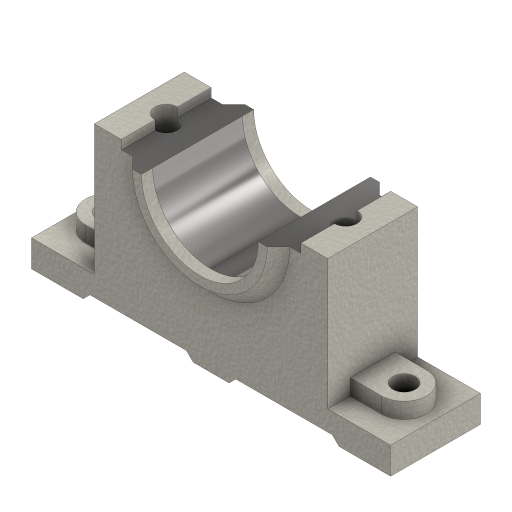
# Autodesk Inventor part: Part039. Lower halg bearing
Saved by Autodesk Inventor 2023.2 (Build 272271030, 271C)
## iProperties
Created: 2023-11-29
Part Number: Part039. Lower halg bearing
Material: Steel, Carbon
Document SubType Name: Modeling
Designer: User
Mass: 237.054 g
Surface Area: 100.472 cm^2
Volume: 30.198 cm^3
Density: 7.85 g/cm^3
Appearance: Steel - Cast
Author: User
Autodesk Inventor part; units mm, degrees
ref_plane "YZ Plane" through (0, 0, 0) normal (1, 0, 0) x (0, 1, 0)
ref_plane "XZ Plane" through (0, 0, 0) normal (0, 1, 0) x (-1, 0, 0)
ref_plane "XY Plane" through (0, 0, 0) normal (0, 0, 1) x (1, 0, 0)
sketch "Sketch1" plane through (0, 0, 0) normal (0, 0, 1) x (1, 0, 0)
  line L0 (0, 0) -> (0, 35) construction
  line L1 (0, 0) -> (-4, 0)
  line L2 (-4, 0) -> (-5.5, 1.5)
  line L3 (-5.5, 1.5) -> (-27, 1.5)
  line L4 (-27, 1.5) -> (-28.5, 0)
  line L5 (-28.5, 0) -> (-40, 0)
  line L6 (-40, 0) -> (-40, 6)
  line L7 (-40, 6) -> (-26, 6)
  line L8 (-26, 6) -> (-26, 35)
  line L9 (-26, 35) -> (-20, 35)
  line L10 (-20, 35) -> (-20, 33)
  line L11 (-20, 33) -> (-13.0111, 33)
  arc A0 (-13.0111, 33) -> (0, 20) centre (-0.0111, 33) ccw
  line L12 (0, 0) -> (4, 0)
  line L13 (4, 0) -> (5.5, 1.5)
  line L14 (5.5, 1.5) -> (27, 1.5)
  line L15 (27, 1.5) -> (28.5, 0)
  line L16 (28.5, 0) -> (40, 0)
  line L17 (40, 0) -> (40, 6)
  line L18 (40, 6) -> (26, 6)
  line L19 (26, 6) -> (26, 35)
  line L20 (26, 35) -> (20, 35)
  line L21 (20, 35) -> (20, 33)
  line L22 (20, 33) -> (13.0111, 33)
  arc A1 (0, 20) -> (13.0111, 33) centre (0.0111, 33) ccw
  dimension "d0" = 35
  dimension "d1" = 45
  dimension "d2" = 45
  dimension "d3" = 24.5
  dimension "d4" = 1.5
  dimension "d5" = 8
  dimension "d6" = 6
  dimension "d7" = 13
  dimension "d8" = 40
  dimension "d9" = 52
  dimension "d10" = 2
  dimension "d11" = 80
  dimension "d12" = 26.9889
  constraints: 46 end point, 12 symmetric about line, 8 point on line, 6 perpendicular, 4 point on circle, 2 centre point, 1 horizontal, 1 parallel, 1 vertical, 1 other
  measures "d0" distance of L0.start L0.end
  measures "d1" angle of L5 L4
  measures "d2" angle of L3 L2
  measures "d3" distance of L1.end L4.end
  measures "d4" distance between parallel lines of L1 L3
  measures "d5" distance of L12.end L1.end
  measures "d6" distance between parallel lines of L16 L18
  measures "d7" radius of A1
  measures "d8" distance between parallel lines of L21 L10
  measures "d9" distance between parallel lines of L19 L8
  measures "d10" distance between parallel lines of L11 L9
  measures "d11" distance between parallel lines of L17 L6
  measures "d12" distance from line of L22.end L17
extrude "Extrusion1" add sketch "Sketch1" along normal mid plane 20
sketch "Sketch2" plane through (26, 6, 10) normal (0, 1, 0) x (1, 0, 0)
  line L0 (0, 20) -> (0, 0) projected
  line L1 (0, 20) -> (0, 0) projected
  line L2 (0, 15) -> (7, 15)
  arc A0 (7, 5) -> (7, 15) centre (7, 10) ccw
  line L3 (7, 5) -> (0, 5)
  line L4 (-26, 20) -> (-26, 0) projected
  point P0 (-26, 10)
  point P1 (-26, 10)
  point P2 (-26, 10)
  dimension "d15" = 5
  dimension "d16" = 33
  constraints: 4 end point, 2 midpoint, 2 point on circle, 2 point on line, 2 tangent, 1 centre point, 1 horizontal, 1 horizontal alignment, 1 parallel
  measures "d15" radius of A0
  measures "d16" distance of point (-26, 10) A0.centre
extrude "Extrusion2" add sketch "Sketch2" along normal blind 3.5
sketch "Sketch3" plane through (26, 9.5, 10) normal (0, 1, 0) x (1, 0, 0)
  arc A0 (7, 5) -> (7, 15) centre (7, 10) ccw projected
  point P0 (-26, 10)
  constraints: 1 coincident
hole "Hole1" at (33, 9.5, 0) direction (0, -1, 0) diameter 5 end through all
mirror "Mirror1" about plane through (0, 0, 0) normal (1, 0, 0) of "Extrusion2", "Hole1"
sketch "Sketch4" plane through (-20, 33, 10) normal (0, 1, 0) x (1, 0, 0)
  line L0 (6.9889, 0) -> (0, 0) projected
  line L1 (6.9889, 0) -> (6.9889, -2.5)
  line L2 (6.9889, -2.5) -> (5, -2.5)
  line L3 (5, -2.5) -> (2.5, 0)
  line L4 (20, 24.7399) -> (20, -8.4394) projected
  point P0 (20, 10)
  dimension "d26" = 30
  dimension "d27" = 45
  dimension "d28" = 12.5
  constraints: 6 end point, 1 perpendicular, 1 point on line, 1 vertical
  measures "d26" diameter of L2.end L4
  measures "d27" angle of L3 L0
  measures "d28" distance from line of L2 point (20, 10)
revolve "Revolution1" add sketch "Sketch4" angle 180 about axis through (0, 33, -10) along (0, 0, 1)
mirror "Mirror2" about plane through (0, 0, 0) normal (0, 0, 1) of "Revolution1"
sketch "Sketch5" plane through (-27, 1.5, 10) normal (0, -1, 0) x (1, 0, 0)
  line L0 (47, -10) -> (7, -10) construction
  point P0 (27, -10)
  point P1 (27, -10)
  dimension "d30" = 40
  constraints: 2 end point, 1 coincident, 1 horizontal, 1 midpoint
  measures "d30" distance of L0.end L0.start
hole "Hole2" at (20, 1.5, 0) at (-20, 1.5, 0) direction (0, 1, 0) diameter 5 end through all counterbore diameter 13 counterbore depth 5
body "Solid1"
